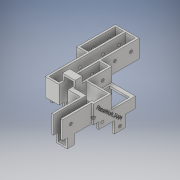
# Autodesk Inventor part: Gear Train Chassis Version 2
Saved by Autodesk Inventor 2017 (Build 210142000, 142)
## iProperties
Created: 2019-11-21
Part Number: Gear Train Chassis Version 2
Material: Generic
Document SubType Name: Modeling
Designer: asadb
Density: 1 g/cm^3
Appearance: Default
Author: asadb
Autodesk Inventor part; units mm, degrees
note: some values were not read from the file. Chosen so that the rebuilt part matches the saved one: direction of "Emboss1".
ref_plane "YZ Plane" through (0, 0, 0) normal (1, 0, 0) x (0, 1, 0)
sketch "Sketch1" plane through (0, 0, 0) normal (0, 1, 0) x (-1, 0, 0)
  line L0 (0, 84.0002) -> (-10, 84.0002)
  line L1 (-10, 84.0002) -> (-10, 76)
  line L2 (-10, 76) -> (-74.5, 76)
  line L3 (-74.5, 76) -> (-74.5, 65.5)
  line L4 (-74.5, 65.5) -> (-91, 65.5)
  line L5 (-91, 65.5) -> (-91, 36)
  line L6 (-91, 36) -> (-69, 36)
  line L7 (-69, 36) -> (-69, 6)
  line L8 (-69, 6) -> (-25, 6)
  line L9 (-25, 6) -> (-25, 0)
  line L10 (-25, 0) -> (0, 0)
  line L11 (0, 16.033) -> (32, 16.033)
  line L12 (32, 16.033) -> (32, 2.033)
  line L13 (32, 2.033) -> (0, 2.033)
  line L14 (0, 0) -> (0, 2.033)
  line L15 (0, 16.033) -> (0, 84.0002)
  point P0 (0, 0)
  point P1 (0, 0)
  dimension "d0" = 84.0002
  dimension "d1" = 25
  dimension "d2" = 6
  dimension "d3" = 44
  dimension "d4" = 30
  dimension "d5" = 29.5
  dimension "d6" = 22
  dimension "d7" = 16.5
  dimension "d8" = 64.5
  dimension "d9" = 76
  dimension "d17" = 2.033
  dimension "d18" = 14
  dimension "d19" = 32
  dimension "d20" = 2.033
  dimension "d21" = 32
  dimension "d22" = 84.0002
  constraints: 32 end point, 13 perpendicular, 2 vertical, 1 horizontal, 1 parallel, 1 other
  measures "d0" distance of L0.start L10.end
  measures "d1" distance of L9.end L10.end
  measures "d2" distance of L9.end L8.end
  measures "d3" distance of L7.end L8.end
  measures "d4" distance of L6.end L7.end
  measures "d5" distance of L4.end L5.end
  measures "d6" distance of L5.end L6.end
  measures "d7" distance of L3.end L4.end
  measures "d8" distance of L1.end L2.end
  measures "d9" distance between parallel lines of L2 L10
  measures "d17" distance from line of point (0, 0) L13
  measures "d18" distance of L11.end L12.end
  measures "d19" distance of L11.start L11.end
  measures "d20" distance of L10.end L13.end
  measures "d21" distance from line of point (0, 0) L12
  measures "d22" distance from line of point (0, 0) L0
surface extrude "ExtrusionSrf1" sketch "Sketch1" along normal blind 30 shown no curves L1 L2 L3 L4 L5 L6 L7 L8 L9 L10 L14 L13 L12 L11 L15 L0
sketch "Sketch2" plane through (0, 0, 0) normal (0, 1, 0) x (-1, 0, 0)
  line L0 (-74.5, 76) -> (-74.5, 65.5) projected
  line L1 (-0.8, 0.8) -> (-21.1, 0.8)
  line L2 (-21.1, 0.8) -> (-21.1, 26.9714)
  line L3 (-21.1, 26.9714) -> (-47.7, 26.9714)
  line L4 (-47.7, 26.9714) -> (-47.7, 39.0002)
  line L5 (-74.5, 65.5) -> (-91, 65.5) projected
  line L6 (-90.2, 65.5) -> (-74.5, 65.5)
  line L7 (-25, 0) -> (0, 0) projected
  line L8 (-0.8, 15.233) -> (31.2, 15.233)
  line L9 (31.2, 2.833) -> (-0.8, 2.833)
  line L10 (-0.8, 2.833) -> (-0.8, 0.8)
  line L11 (32, 16.033) -> (0, 16.033) projected
  line L12 (32, 2.033) -> (32, 16.033) projected
  line L13 (0, 2.033) -> (32, 2.033) projected
  line L14 (0, 0) -> (0, 2.033) projected
  line L15 (-25, 6) -> (-25, 0) projected
  line L16 (0, 16.033) -> (0, 84.0002) projected
  line L17 (5.242, 5.033) -> (29, 5.033)
  line L18 (29, 13.033) -> (6.042, 13.033)
  line L19 (-18.9, 3) -> (-3.8, 3)
  line L20 (-18.9, 20.868) -> (-18.9, 3)
  line L21 (5.242, 5.033) -> (-3.8, 5.033)
  line L22 (6.042, 13.033) -> (-5.6, 13.033)
  line L23 (-3.8, 3) -> (-3.8, 5.033)
  line L24 (-5.6, 13.033) -> (-5.6, 20.868)
  line L25 (31.2, 15.233) -> (31.2, 13.033)
  line L26 (31.2, 5.033) -> (31.2, 2.833)
  line L27 (29, 13.033) -> (31.2, 13.033)
  line L28 (29, 5.033) -> (31.2, 5.033)
  line L29 (23, 13.033) -> (23, 5.033) construction
  line L30 (-10.9, 3) -> (-10.9, 52.2501) construction
  line L31 (-81, 65.5) -> (-81, 76) construction
  line L32 (-91, 65.5) -> (-91, 36) construction
  line L33 (-88, 63.3) -> (-63.0024, 63.3)
  line L34 (-63.0024, 39.0002) -> (-88, 39.0002)
  line L35 (-91, 36) -> (-69, 36) construction
  line L36 (-45.5, 39.0002) -> (-45.5, 29.1714)
  line L37 (-45.5, 29.1714) -> (-21.6831, 29.1714)
  line L38 (-18.9, 26.9714) -> (-18.9, 20.868)
  line L39 (-37.5, 52.2501) -> (-37.5, 29.1714) construction
  line L40 (-30.5, 29.1714) -> (-30.5, 52.2501) construction
  line L41 (0, 84.0002) -> (-10, 84.0002) projected
  line L42 (-3, 41.2002) -> (-88, 41.2002)
  line L43 (-81, 65.5) -> (-81, 41.2002) construction
  line L44 (-81, 39.0002) -> (-81, 39.0002) construction
  line L45 (-63, 63.3) -> (-63, 41.2002) construction
  line L46 (-45.5, 39.0002) -> (-45.5, 39.0002) construction
  line L47 (-90.2, 39.0002) -> (-90.2, 65.5)
  line L48 (-88, 39.0002) -> (-90.2, 39.0002)
  line L49 (-3, 52.2501) -> (-3, 41.2002)
  line L50 (-5.6, 26.9714) -> (-5.6, 20.868)
  line L51 (-69, 36) -> (-69, 6) projected
  line L52 (-3, 39.0002) -> (-0.8, 39.0002)
  line L53 (-21.6831, 29.1714) -> (-3, 29.1714)
  line L54 (-18.9, 26.9714) -> (-5.6, 26.9714)
  line L55 (-3, 29.1714) -> (-0.8, 29.1714)
  line L56 (-0.8, 29.1714) -> (-0.8, 15.233)
  line L57 (-69, 6) -> (-25, 6) projected
  line L58 (-88, 52.2501) -> (-3, 52.2501)
  line L59 (-49, 63.3) -> (-49, 54.4501)
  line L60 (-46.8, 63.3) -> (-46.8, 54.4501)
  line L61 (-46.8, 63.3) -> (-46.8, 65.5)
  line L62 (-74.5, 65.5) -> (-46.8, 65.5)
  line L63 (-63, 63.3) -> (-49, 63.3)
  line L64 (-0.8, 54.4501) -> (-0.8, 39.0002)
  line L65 (-3, 54.4501) -> (-0.8, 54.4501)
  line L66 (-88, 54.4501) -> (-49, 54.4501)
  line L67 (-46.8, 54.4501) -> (-3, 54.4501)
  line L68 (-88, 41.2002) -> (-88, 52.2501)
  line L69 (-88, 54.4501) -> (-88, 63.3)
  line L70 (-3, 39.0002) -> (-45.5, 39.0002)
  line L71 (-47.7, 39.0002) -> (-88, 39.0002)
  dimension "d14" = 0.8
  dimension "d23" = 0.8
  dimension "d25" = 0.8
  dimension "d26" = 0.8
  dimension "d33" = 3
  dimension "d35" = 3
  dimension "d36" = 3
  dimension "d37" = 5.6
  dimension "d38" = 3
  dimension "d43" = 0.8
  dimension "d44" = 0.8
  dimension "d45" = 9
  dimension "d53" = 10
  dimension "d60" = 2.2
  dimension "d65" = 2.2
  dimension "d67" = 26.6
  dimension "d68" = 30.5
  dimension "d71" = 0.8
  dimension "d74" = 8
  dimension "d75" = 8
  dimension "d76" = 2.2
  dimension "d79" = 21.3
  dimension "d80" = 20.9714
  dimension "d82" = 2.2
  dimension "d83" = 14
  dimension "d84" = 18
  dimension "d85" = 2.2
  dimension "d86" = 0.8
  dimension "d87" = 29.5501
  dimension "d88" = 2.2
  dimension "d89" = 4.8
  dimension "d90" = 2.2
  dimension "d91" = 2.2
  dimension "d92" = 2.2
  dimension "d93" = 2.2
  dimension "d94" = 2.2
  dimension "d95" = 40.3
  dimension "d96" = 85
  dimension "d97" = 42.5
  dimension "d98" = 11.0499
  dimension "d99" = 2.2
  constraints: 116 end point, 36 perpendicular, 20 point on line, 12 parallel, 8 horizontal, 5 collinear, 3 vertical
  measures "d14" distance between parallel lines of L7 L1
  measures "d23" distance between parallel lines of L11 L8
  measures "d25" distance between parallel lines of L13 L9
  measures "d26" distance between parallel lines of L14 L10
  measures "d33" distance between parallel lines of L7 L19
  measures "d35" distance between parallel lines of L11 L18
  measures "d36" distance between parallel lines of L13 L17
  measures "d37" distance between parallel lines of L16 L24
  measures "d38" distance between parallel lines of L10 L23
  measures "d43" distance between parallel lines of L12 L25
  measures "d44" distance between parallel lines of L12 L26
  measures "d45" distance between parallel lines of L12 L29
  measures "d53" distance between parallel lines of L32 L31
  measures "d60" distance between parallel lines of L6 L33
  measures "d65" distance between parallel lines of L4 L36
  measures "d67" distance between parallel lines of L39 L30
  measures "d68" distance between parallel lines of L16 L40
  measures "d71" distance from line of L5.end L47
  measures "d74" distance between parallel lines of L36 L39
  measures "d75" distance between parallel lines of L38 L30
  measures "d76" distance between parallel lines of L2 L20
  measures "d79" distance between parallel lines of L51 L4
  measures "d80" distance between parallel lines of L57 L3
  measures "d82" distance between parallel lines of L60 L59
  measures "d83" distance between parallel lines of L45 L59
  measures "d84" distance between parallel lines of L43 L45
  measures "d85" distance between parallel lines of L49 L64
  measures "d86" distance between parallel lines of L16 L64
  measures "d87" distance between parallel lines of L41 L65
  measures "d88" distance between parallel lines of L3 L37
  measures "d89" distance between parallel lines of L50 L56
  measures "d90" distance between parallel lines of L58 L66
  measures "d91" distance between parallel lines of L47 L69
  measures "d92" distance between parallel lines of L71 L42
  measures "d93" distance between parallel lines of L70 L42
  measures "d94" distance between parallel lines of L58 L67
  measures "d95" distance of L4.end L48.start
  measures "d96" distance of L42.start L42.end
  measures "d97" distance of L52.start L36.start
  measures "d98" distance of L42.end L58.start
  measures "d99" distance between parallel lines of L53 L54
extrude "Extrusion1" add sketch "Sketch2" along normal blind 20
sketch "Sketch3" plane through (0, 0, 0) normal (0, -1, 0) x (1, 0, 0)
  line L0 (88, 63.3) -> (49, 63.3)
  line L1 (49, 63.3) -> (49, 54.4501)
  line L2 (49, 54.4501) -> (88, 54.4501)
  line L3 (88, 54.4501) -> (88, 63.3)
  line L4 (46.8, 65.5) -> (90.2, 65.5) projected
  line L5 (90.2, 65.5) -> (90.2, 39.0002) projected
  line L6 (3, 52.2501) -> (88, 52.2501) projected
  line L7 (46.8, 54.4501) -> (46.8, 65.5) projected
  point P0 (0, 0)
  dimension "d102" = 2.2
  dimension "d103" = 2.2
  dimension "d104" = 2.2
  dimension "d105" = 2.2
  constraints: 8 end point, 2 parallel, 1 horizontal, 1 perpendicular
  measures "d102" distance between parallel lines of L4 L0
  measures "d103" distance between parallel lines of L5 L3
  measures "d104" distance between parallel lines of L6 L2
  measures "d105" distance between parallel lines of L7 L1
extrude "Extrusion2" cut sketch "Sketch3" against normal blind 20
ref_plane "Work Plane1" through (10.9, 0, 29.1714) normal (-1, 0, 0) x (0, 0, 1)
sketch "Sketch4" plane through (10.9, 0, 29.1714) normal (-1, 0, 0) x (0, 0, 1)
  line L0 (9.6527, -4.76) -> (-0.0402, -4.76) construction
  line L1 (0, 0) -> (0, 20) construction
  line L2 (9.8288, 20) -> (25.2787, 20) construction
  line L3 (-13.9384, 0) -> (0, 0) construction
  line L4 (10.9288, -5.86) -> (-1.1, -5.86)
  line L5 (9.8288, 0) -> (9.8288, 20) projected
  line L6 (10.9288, -5.86) -> (10.9288, 0)
  line L7 (-1.1, -5.86) -> (-1.1, 0)
  point P0 (-29.1714, 0)
  point P1 (4.9145, 22.24)
  dimension "d109" = 4.9145
  dimension "d110" = 2.24
  dimension "d111" = 27
  dimension "d112" = 9.6929
  dimension "d113" = 4.9547
  dimension "d114" = 1.1
  dimension "d115" = 1.1
  dimension "d116" = 28.1
  constraints: 8 end point, 1 horizontal, 1 parallel, 1 perpendicular, 1 point on line, 1 vertical
  measures "d109" distance from line of L1 point (4.915, 22.24)
  measures "d110" distance from line of L2 point (4.915, 22.24)
  measures "d111" distance from line of point (4.915, 22.24) L0
  measures "d112" distance of L0.start L0.end
  measures "d113" horizontal distance of L0.end point (4.915, 22.24)
  measures "d114" horizontal distance of L1.start L4.end
  measures "d115" distance from line of L5 L4.start
  measures "d116" distance from line of point (4.915, 22.24) L4
sketch "Sketch6" plane through (0, 0, 0) normal (0, -1, 0) x (1, 0, 0)
  line L0 (14.8, 41.2002) -> (6.8, 41.2002)
  line L1 (6.8, 41.2002) -> (6.8, 39.0002)
  line L2 (6.8, 39.0002) -> (14.8, 39.0002)
  line L3 (14.8, 39.0002) -> (14.8, 41.2002)
  line L4 (88, 41.2002) -> (3, 41.2002) projected
  line L5 (0.8, 39.0002) -> (0.8, 54.4501) projected
  point P0 (0, 0)
  dimension "d117" = 2.2
  dimension "d118" = 0
  dimension "d119" = 8
  dimension "d120" = 6
  constraints: 8 end point, 2 parallel, 1 horizontal, 1 perpendicular
  measures "d117" distance of L1.end L0.end
  measures "d118" distance between parallel lines of L4 L0
  measures "d119" distance between parallel lines of L1 L3
  measures "d120" distance between parallel lines of L5 L1
sweep "Sweep1" add profiles "Sketch6" path "Sketch4" path curves L6 L4 L7
sketch "Sketch7" plane through (0.8, 0, 2.833) normal (0, 0, -1) x (-1, 0, 0)
  line L0 (32, 0) -> (32, 20) projected
  line L1 (32, 0) -> (-3, 0) projected
  point P0 (0.8, 0)
  point P1 (23, 8.5)
  dimension "d123" = 9
  dimension "d124" = 8.5
  measures "d123" distance from line of point (23, 8.5) L0
  measures "d124" distance from line of L1 point (23, 8.5)
ref_plane "Work Plane2" through (-22.2, 0, 13.033) normal (-1, 0, 0) x (0, 0, 1)
sketch "Sketch8" plane through (-22.2, 0, 13.033) normal (-1, 0, 0) x (0, 0, 1)
  line L0 (0, 0) -> (0, 20) projected
  line L1 (0, 0) -> (2.2, 0) projected
  line L2 (1.1, 29.5) -> (-9.1, 29.5)
  line L3 (-10.2, 0) -> (-10.2, 20) projected
  line L4 (2.2, 0) -> (2.2, 20) projected
  line L5 (1.1, 29.5) -> (1.1, 20)
  line L6 (0, 20) -> (2.2, 20) projected
  line L7 (-9.1, 29.5) -> (-9.1, 20)
  line L8 (-8, 20) -> (-10.033, 20) projected
  line L9 (-10.2, 20) -> (-8, 20) projected
  point P0 (-13.033, 0)
  point P1 (-4, 8.5)
  dimension "d126" = 4
  dimension "d127" = 8.5
  dimension "d128" = 1.1
  dimension "d129" = 1.1
  dimension "d130" = 21
  constraints: 6 end point, 2 perpendicular, 1 horizontal, 1 midpoint, 1 point on line
  measures "d126" distance from line of L0 point (-4, 8.5)
  measures "d127" distance from line of L1 point (-4, 8.5)
  measures "d128" distance from line of L3 L2.end
  measures "d129" distance from line of L4 L2.start
  measures "d130" distance from line of point (-4, 8.5) L2
sketch "Sketch9" plane through (0, 20, 0) normal (0, 1, 0) x (1, 0, 0)
  line L0 (-26.2, -15.233) -> (-18.2, -15.233)
  line L1 (-18.2, -15.233) -> (-18.2, -13.033)
  line L2 (-18.2, -13.033) -> (-26.2, -13.033)
  line L3 (-26.2, -13.033) -> (-26.2, -15.233)
  line L4 (-31.2, -15.233) -> (0.8, -15.233) projected
  line L5 (5.6, -13.033) -> (-31.2, -13.033) projected
  line L6 (-31.2, -13.033) -> (-31.2, -15.233) projected
  point P0 (0, 0)
  dimension "d131" = 0
  dimension "d132" = 0
  dimension "d134" = 8
  dimension "d135" = 5
  constraints: 8 end point, 2 parallel, 1 horizontal, 1 perpendicular
  measures "d131" distance between parallel lines of L4 L0
  measures "d132" distance between parallel lines of L5 L2
  measures "d134" distance of L1.end L2.end
  measures "d135" distance between parallel lines of L3 L6
sweep "Sweep2" add profiles "Sketch9" path "Sketch8" path curves L5 L2 L7 contours L3 L2 L1 L0
sketch "Sketch10" plane through (90.2, 0, 39.0002) normal (0, 0, -1) x (-1, 0, 0)
  line L0 (0, 0) -> (0, 20) projected
  line L1 (0, 0) -> (42.5, 0) projected
  line L2 (44.7, 0) -> (75.4, 0) projected
  point P0 (90.2, 0)
  point P1 (9.2, 8.5)
  point P2 (27.2, 8.5)
  point P3 (52.7, 8.5)
  dimension "d138" = 9.2
  dimension "d139" = 8.5
  dimension "d140" = 18
  dimension "d141" = 8.5
  dimension "d143" = 25.5
  dimension "d144" = 8.5
  measures "d138" distance from line of L0 point (9.2, 8.5)
  measures "d139" distance from line of L1 point (9.2, 8.5)
  measures "d140" distance of point (9.2, 8.5) point (27.2, 8.5)
  measures "d141" distance from line of L1 point (27.2, 8.5)
  measures "d143" distance of point (27.2, 8.5) point (52.7, 8.5)
  measures "d144" distance from line of L2 point (52.7, 8.5)
hole "Hole1" at (63, 8.5, 39.0002) at (81, 8.5, 39.0002) direction (0, 0, 1) diameter 3.302 end through all
sketch "Sketch11" plane through (47.7, 0, 26.9714) normal (0, 0, -1) x (-1, 0, 0)
  line L0 (32.9, 0) -> (2.2, 0) projected
  line L1 (-42.5, 0) -> (-42.5, 20) projected
  point P0 (47.7, 0)
  point P1 (10.2, 8.5)
  dimension "d152" = 8.5
  dimension "d153" = 52.7
  measures "d152" distance from line of L0 point (10.2, 8.5)
  measures "d153" distance from line of L1 point (10.2, 8.5)
hole "Hole2" at (37.5, 8.5, 26.9714) direction (0, 0, 1) diameter 3.302 end through all
hole "Hole3" at (-22.2, 8.5, 2.833) direction (0, 0, 1) diameter 3.302 end through all
sketch "Sketch12" plane through (0, 20, 0) normal (0, 1, 0) x (1, 0, 0)
  line L0 (6.8, -52.2501) -> (14.8, -52.2501)
  line L1 (14.8, -52.2501) -> (14.8, -54.4501)
  line L2 (14.8, -54.4501) -> (6.8, -54.4501)
  line L3 (6.8, -54.4501) -> (6.8, -52.2501)
  line L4 (3, -52.2501) -> (88, -52.2501) projected
  line L5 (0.8, -39.0002) -> (0.8, -54.4501) projected
  line L6 (6.8, -39.0002) -> (14.8, -39.0002)
  line L7 (14.8, -39.0002) -> (14.8, -41.2002)
  line L8 (14.8, -41.2002) -> (6.8, -41.2002)
  line L9 (6.8, -41.2002) -> (6.8, -39.0002)
  line L10 (6.8, -26.9714) -> (14.8, -26.9714)
  line L11 (14.8, -26.9714) -> (14.8, -29.1714)
  line L12 (14.8, -29.1714) -> (6.8, -29.1714)
  line L13 (6.8, -29.1714) -> (6.8, -26.9714)
  line L14 (6.8, -0.8) -> (14.8, -0.8)
  line L15 (14.8, -0.8) -> (14.8, -3)
  line L16 (14.8, -3) -> (6.8, -3)
  line L17 (6.8, -3) -> (6.8, -0.8)
  line L18 (3, -41.2002) -> (88, -41.2002) construction
  line L19 (18.9, -26.9714) -> (5.6, -26.9714) construction
  line L20 (3.8, -3) -> (18.9, -3) construction
  point P0 (0, 0)
  dimension "d168" = 8
  dimension "d169" = 2.2
  dimension "d170" = 0
  dimension "d171" = 6
  dimension "d172" = 8
  dimension "d173" = 2.2
  dimension "d174" = 8
  dimension "d175" = 2.2
  dimension "d176" = 8
  dimension "d177" = 2.2
  dimension "d178" = 0
  dimension "d179" = 0
  dimension "d180" = 0
  constraints: 32 end point, 8 parallel, 4 horizontal, 4 perpendicular, 3 collinear
  measures "d168" distance of L1.end L2.end
  measures "d169" distance of L0.end L1.end
  measures "d170" distance between parallel lines of L4 L0
  measures "d171" distance between parallel lines of L5 L3
  measures "d172" distance of L7.end L8.end
  measures "d173" distance of L6.end L7.end
  measures "d174" distance of L11.end L12.end
  measures "d175" distance of L10.end L11.end
  measures "d176" distance of L15.end L16.end
  measures "d177" distance of L14.end L15.end
  measures "d178" distance between parallel lines of L18 L8
  measures "d179" distance between parallel lines of L19 L10
  measures "d180" distance between parallel lines of L20 L16
extrude "Extrusion3" add sketch "Sketch12" along normal blind 7.5
sketch "Sketch15" plane through (0.8, 0, 54.4501) normal (0, 0, 1) x (1, 0, 0)
  circle A0 centre (36.7, 8.5) radius 1.651 construction
  line L0 (36.7, 8.5) -> (10.0336, 22.2441) construction
  line L1 (36.7, 8.5) -> (66.7, 8.5) construction
  point P0 (-0.8, 0)
  dimension "d203" = 30
  dimension "d204" = 152.733
  constraints: 4 end point, 1 coincident, 1 equal length, 1 horizontal
  measures "d203" distance of L0.start L0.end
  measures "d204" angle of L1 L0
hole "Hole6" at (10.8336, 22.2441, 54.4501) direction (0, 0, -1) diameter 3.302 end through all
sketch "Sketch16" plane through (21.1, 0, 0.8) normal (0, 0, -1) x (-1, 0, 0)
  circle A0 centre (10.2664, 22.2441) radius 1.651 construction
  line L0 (10.2664, 22.2441) -> (19.3486, 13.6555) construction
  line L1 (10.2664, 22.2441) -> (22.7664, 22.2441) construction
  circle A1 centre (43.3, 8.5) radius 1.651 projected
  point P0 (21.1, 0)
  dimension "d212" = 12.5
  dimension "d257" = 24.5
  constraints: 4 end point, 1 coincident, 1 equal length, 1 horizontal
  measures "d212" distance of L0.start L0.end
  measures "d257" distance of A1.centre point (19.349, 13.655)
hole "Hole7" at (1.7514, 13.6555, 0.8) direction (0, 0, 1) diameter 3.302 depth 16.533 tip angle 118
sketch "Sketch17" plane through (21.1, 0, 0.8) normal (0, 0, -1) x (-1, 0, 0)
  circle A0 centre (-16.4, 8.5) radius 1.651 construction
  line L0 (-16.4, 8.5) -> (-9.4008, 35.9992) construction
  line L1 (-16.4, 8.5) -> (11.9759, 8.5) construction
  circle A1 centre (10.2664, 22.2441) radius 1.651 construction
  point P0 (21.1, 0)
  dimension "d221" = 75.72
  dimension "d222" = 24
  constraints: 4 end point, 1 coincident, 1 equal length, 1 horizontal
  measures "d221" angle of L1 L0
  measures "d222" distance of A1.centre L0.end
sketch "Sketch18" plane through (14.8, 20, 3) normal (1, 0, 0) x (0, 0, -1)
  line L0 (2.2, 0) -> (2.2, 7.5) projected
  line L1 (0, 0) -> (0, 7.5) projected
  line L2 (2.2, 0) -> (0, 0)
  line L3 (0, 0) -> (0, 7.5)
  line L4 (0, 7.5) -> (2.2, 7.5)
  line L5 (2.2, 7.5) -> (2.2, 0)
  line L6 (-23.9714, 0) -> (-26.1714, 0) projected
  line L7 (-26.1714, 0) -> (-26.1714, 7.5) projected
  line L8 (-23.9714, 0) -> (-26.1714, 0)
  line L9 (-26.1714, 0) -> (-26.1714, 7.5)
  line L10 (-26.1714, 7.5) -> (-23.9714, 7.5)
  line L11 (-23.9714, 7.5) -> (-23.9714, 0)
  point P0 (3, -20)
  constraints: 16 end point, 4 parallel, 2 horizontal, 2 perpendicular
extrude "Extrusion4" add sketch "Sketch18" along normal up to surface (32.9 mm away)
sketch "Sketch19" plane through (21.1, 0, 26.9714) normal (1, 0, 0) x (0, 0, -1)
  line L0 (23.9714, 20) -> (26.1714, 20) projected
  line L1 (0, 0) -> (0, 20) projected
  line L2 (26.1714, 20) -> (0, 20)
  line L3 (0, 20) -> (0, 17.8)
  line L4 (0, 17.8) -> (26.1714, 17.8)
  line L5 (26.1714, 17.8) -> (26.1714, 20)
  point P0 (26.9714, 0)
  dimension "d225" = 2.2
  constraints: 8 end point, 2 parallel, 1 horizontal, 1 perpendicular, 1 point on line
  measures "d225" distance of L3.end L2.end
extrude "Extrusion5" add sketch "Sketch19" along normal up to surface (26.6 mm away)
sketch "Sketch20" plane through (0, 27.5, 0) normal (0, 1, 0) x (1, 0, 0)
  line L0 (6.8, -0.8) -> (47.7, -0.8) projected
  line L1 (6.8, -3) -> (47.7, -3) projected
  line L2 (24.2, -0.8) -> (36.2, -0.8)
  line L3 (36.2, -0.8) -> (36.2, -3)
  line L4 (36.2, -3) -> (24.2, -3)
  line L5 (24.2, -3) -> (24.2, -0.8)
  line L6 (47.7, -3) -> (47.7, -0.8) projected
  line L7 (6.8, -29.1714) -> (47.7, -29.1714) projected
  line L8 (24.2, -29.1714) -> (36.2, -29.1714)
  line L9 (36.2, -29.1714) -> (36.2, -26.9714)
  line L10 (36.2, -26.9714) -> (24.2, -26.9714)
  line L11 (24.2, -26.9714) -> (24.2, -29.1714)
  point P0 (0, 0)
  dimension "d228" = 12
  dimension "d229" = 11.5
  dimension "d230" = 12
  dimension "d231" = 2.2
  dimension "d232" = 0
  constraints: 16 end point, 4 parallel, 3 point on line, 2 horizontal, 2 perpendicular
  measures "d228" distance between parallel lines of L3 L5
  measures "d229" distance between parallel lines of L6 L3
  measures "d230" distance of L10.end L9.end
  measures "d231" distance of L9.end L8.end
  measures "d232" distance between parallel lines of L11 L5
extrude "Extrusion6" add sketch "Sketch20" along normal blind 13 contours L0 L3 L1 L5 | L11 L10 L9 L7
hole "Hole8" at (30.5008, 35.9992, 0.8) direction (0, 0, 1) diameter 3.302 end through all
sketch "Sketch21" plane through (47.7, 0, 39.0002) normal (1, 0, 0) x (0, 0, -1)
  line L0 (36.0002, 20) -> (36.0002, 27.5) projected
  line L1 (38.2002, 17.8) -> (12.0288, 17.8) projected
  line L2 (36.0002, 20) -> (12.0288, 20)
  line L3 (12.0288, 20) -> (12.0288, 17.8)
  line L4 (12.0288, 17.8) -> (36.0002, 17.8)
  line L5 (36.0002, 17.8) -> (36.0002, 20)
  point P0 (39.0002, 0)
  constraints: 8 end point, 2 parallel, 1 horizontal, 1 perpendicular
extrude "Extrusion7" cut sketch "Sketch21" against normal blind 29
sketch "Sketch23" plane through (47.7, 0, 39.0002) normal (1, 0, 0) x (0, 0, -1)
  line L0 (38.2002, 27.5) -> (38.2002, 17.8) projected
  line L1 (12.0288, 0) -> (12.0288, 17.8) projected
  line L2 (38.2002, 17.8) -> (12.0288, 17.8)
  line L3 (12.0288, 17.8) -> (12.0288, 15.6)
  line L4 (12.0288, 15.6) -> (38.2002, 15.6)
  line L5 (38.2002, 15.6) -> (38.2002, 17.8)
  point P0 (39.0002, 0)
  dimension "d245" = 2.2
  constraints: 8 end point, 2 parallel, 1 horizontal, 1 perpendicular, 1 point on line
  measures "d245" distance of L3.end L2.end
extrude "Extrusion8" add sketch "Sketch23" against normal blind 4.4167
sketch "Sketch24" plane through (21.1, 17.8, 0.8) normal (0, -1, 0) x (1, 0, 0)
  line L0 (0, 0) -> (0, 2.2) projected
  line L1 (22.1833, 0) -> (22.1833, 26.1714) projected
  line L2 (0, 0) -> (22.1833, 0)
  line L3 (22.1833, 0) -> (22.1833, 2.2)
  line L4 (22.1833, 2.2) -> (0, 2.2)
  line L5 (0, 2.2) -> (0, 0)
  point P0 (-21.1, -0.8)
  dimension "d248" = 2.2
  constraints: 8 end point, 2 parallel, 1 horizontal, 1 perpendicular, 1 point on line
  measures "d248" distance of L3.end L2.end
extrude "Extrusion9" add sketch "Sketch24" along normal blind 2.2
sketch "Sketch25" plane through (21.1, 0, 26.9714) normal (1, 0, 0) x (0, 0, -1)
  line L0 (0, 0) -> (0, 17.8) projected
  line L1 (0, 17.8) -> (2.2, 17.8)
  line L2 (2.2, 17.8) -> (2.2, 15.6)
  line L3 (2.2, 15.6) -> (0, 15.6)
  line L4 (0, 15.6) -> (0, 17.8)
  point P0 (26.9714, 0)
  dimension "d251" = 2.2
  dimension "d252" = 2.2
  constraints: 8 end point, 2 parallel, 1 horizontal, 1 perpendicular
  measures "d251" distance of L2.end L3.end
  measures "d252" distance of L1.end L2.end
extrude "Extrusion10" add sketch "Sketch25" along normal up to surface (22.1833 mm away)
sketch "Sketch26" plane through (21.1, 0, 0.8) normal (0, 0, -1) x (-1, 0, 0)
  line L0 (15.1438, 3.2996) -> (-7.5912, 23.6414) construction
  line L1 (-7.5912, 23.6414) -> (-0.9379, 31.0775) construction
  line L2 (-0.9379, 31.0775) -> (21.7972, 10.7357) construction
  line L3 (21.7972, 10.7357) -> (15.1438, 3.2996) construction
  spline S0 degree 2 poles (14.0385, 5.9137) (14.1898, 6.0828) (14.5826, 6.2794) (14.7849, 6.2886) knots 0 0 0 1 2 2 2
  spline S1 degree 2 poles (14.7849, 6.2886) (15.0394, 6.3008) (15.528, 6.111) (15.807, 5.8613) knots 0 0 0 1 2 2 2
  line L4 (15.807, 5.8613) -> (16.1008, 5.5984)
  line L5 (16.1008, 5.5984) -> (16.9708, 6.5708)
  line L6 (16.9708, 6.5708) -> (17.3174, 6.2606)
  line L7 (17.3174, 6.2606) -> (14.9836, 3.6522)
  line L8 (14.9836, 3.6522) -> (14.3284, 4.2385)
  spline S2 degree 2 poles (14.3284, 4.2385) (14.0959, 4.4466) (13.8384, 4.8139) (13.7913, 5.0121) knots 0 0 0 1 2 2 2
  spline S3 degree 2 poles (13.7913, 5.0121) (13.7343, 5.242) (13.8437, 5.696) (14.0385, 5.9137) knots 0 0 0 1 2 2 2
  spline S4 degree 2 poles (14.4094, 5.6009) (14.2883, 5.4656) (14.2036, 5.1837) (14.2419, 5.0352) knots 0 0 0 1 2 2 2
  spline S5 degree 2 poles (14.2419, 5.0352) (14.2752, 4.9065) (14.4553, 4.6654) (14.6181, 4.5198) knots 0 0 0 1 2 2 2
  line L9 (14.6181, 4.5198) -> (14.9055, 4.2626)
  line L10 (14.9055, 4.2626) -> (15.836, 5.3025)
  line L11 (15.836, 5.3025) -> (15.5993, 5.5143)
  spline S6 degree 2 poles (15.5993, 5.5143) (15.3879, 5.7035) (15.0674, 5.8684) (14.9034, 5.8553) knots 0 0 0 1 2 2 2
  spline S7 degree 2 poles (14.9034, 5.8553) (14.7552, 5.8471) (14.5209, 5.7256) (14.4094, 5.6009) knots 0 0 0 1 2 2 2
  line L12 (15.0282, 8.3088) -> (15.358, 8.0138)
  line L13 (15.358, 8.0138) -> (12.9202, 5.2892)
  line L14 (12.9202, 5.2892) -> (12.5904, 5.5842)
  line L15 (12.5904, 5.5842) -> (15.0282, 8.3088)
  spline S8 degree 2 poles (13.7342, 9.5465) (14.2034, 9.1267) (14.2483, 8.1389) (13.8133, 7.6528) knots 0 0 0 1 2 2 2
  spline S9 degree 2 poles (13.8133, 7.6528) (13.3859, 7.1751) (12.3781, 7.0568) (11.9743, 7.418) knots 0 0 0 1 2 2 2
  spline S10 degree 2 poles (11.9743, 7.418) (11.7926, 7.5807) (11.606, 7.9379) (11.6027, 8.1426) knots 0 0 0 1 2 2 2
  spline S11 degree 2 poles (11.6027, 8.1426) (11.5972, 8.3492) (11.7745, 8.7728) (11.9845, 9.0074) knots 0 0 0 1 2 2 2
  line L16 (11.9845, 9.0074) -> (12.1452, 9.1871)
  line L17 (12.1452, 9.1871) -> (13.5001, 7.9748)
  spline S12 degree 2 poles (13.5001, 7.9748) (13.8046, 8.3151) (13.7856, 8.983) (13.4812, 9.2553) knots 0 0 0 1 2 2 2
  spline S13 degree 2 poles (13.4812, 9.2553) (13.3734, 9.3517) (13.1206, 9.4904) (13.002, 9.528) knots 0 0 0 1 2 2 2
  spline S14 degree 2 poles (13.002, 9.528) (12.8754, 9.5651) (12.6867, 9.6008) (12.6162, 9.6029) knots 0 0 0 1 2 2 2
  line L18 (12.6162, 9.6029) -> (12.5972, 9.62)
  line L19 (12.5972, 9.62) -> (12.9187, 9.9793)
  spline S15 degree 2 poles (12.9187, 9.9793) (12.9966, 9.9515) (13.2304, 9.8641) (13.3151, 9.8226) knots 0 0 0 1 2 2 2
  spline S16 degree 2 poles (13.3151, 9.8226) (13.4348, 9.7649) (13.6158, 9.6525) (13.7342, 9.5465) knots 0 0 0 1 2 2 2
  spline S17 degree 2 poles (12.2414, 8.6481) (12.1265, 8.5111) (12.0075, 8.2675) (12.0017, 8.1547) knots 0 0 0 1 2 2 2
  spline S18 degree 2 poles (12.0017, 8.1547) (11.9926, 8.0297) (12.1023, 7.7907) (12.2354, 7.6716) knots 0 0 0 1 2 2 2
  spline S19 degree 2 poles (12.2354, 7.6716) (12.3665, 7.5543) (12.6204, 7.468) (12.7645, 7.476) knots 0 0 0 1 2 2 2
  spline S20 degree 2 poles (12.7645, 7.476) (12.9085, 7.488) (13.1529, 7.608) (13.2751, 7.7233) knots 0 0 0 1 2 2 2
  line L20 (13.2751, 7.7233) -> (12.2414, 8.6481)
  spline S21 degree 2 poles (11.3806, 11.1995) (11.4472, 11.1931) (11.6771, 11.1778) (11.7688, 11.1528) knots 0 0 0 1 2 2 2
  spline S22 degree 2 poles (11.7688, 11.1528) (11.8971, 11.1217) (12.1034, 11.0247) (12.2513, 10.8923) knots 0 0 0 1 2 2 2
  spline S23 degree 2 poles (12.2513, 10.8923) (12.3718, 10.7845) (12.5082, 10.4988) (12.5169, 10.3426) knots 0 0 0 1 2 2 2
  spline S24 degree 2 poles (12.5169, 10.3426) (12.5232, 10.1923) (12.4065, 9.8705) (12.2893, 9.7394) knots 0 0 0 1 2 2 2
  spline S25 degree 2 poles (12.2893, 9.7394) (12.1077, 9.5365) (11.6793, 9.4023) (11.4195, 9.4862) knots 0 0 0 1 2 2 2
  spline S26 degree 2 poles (11.4195, 9.4862) (11.1866, 9.5577) (10.6874, 9.9015) (10.4142, 10.1194) knots 0 0 0 1 2 2 2
  line L21 (10.4142, 10.1194) -> (10.3574, 10.0559)
  spline S27 degree 2 poles (10.3574, 10.0559) (10.2553, 9.9418) (10.1984, 9.7378) (10.2258, 9.6409) knots 0 0 0 1 2 2 2
  spline S28 degree 2 poles (10.2258, 9.6409) (10.2533, 9.544) (10.4124, 9.356) (10.5096, 9.269) knots 0 0 0 1 2 2 2
  spline S29 degree 2 poles (10.5096, 9.269) (10.6238, 9.1668) (10.9929, 8.9584) (11.2058, 8.8858) knots 0 0 0 1 2 2 2
  line L22 (11.2058, 8.8858) -> (11.2248, 8.8688)
  line L23 (11.2248, 8.8688) -> (10.9241, 8.5327)
  spline S30 degree 2 poles (10.9241, 8.5327) (10.8106, 8.5887) (10.4135, 8.8298) (10.2465, 8.9792) knots 0 0 0 1 2 2 2
  spline S31 degree 2 poles (10.2465, 8.9792) (10.0436, 9.1607) (9.8234, 9.4719) (9.7873, 9.6527) knots 0 0 0 1 2 2 2
  spline S32 degree 2 poles (9.7873, 9.6527) (9.7514, 9.8294) (9.8745, 10.1798) (10.039, 10.3637) knots 0 0 0 1 2 2 2
  line L24 (10.039, 10.3637) -> (11.2362, 11.7017)
  line L25 (11.2362, 11.7017) -> (11.5659, 11.4066)
  line L26 (11.5659, 11.4066) -> (11.3806, 11.1995)
  line L27 (11.1347, 10.9247) -> (10.6487, 10.3815)
  spline S33 degree 2 poles (10.6487, 10.3815) (10.7765, 10.2861) (11.1659, 10.0024) (11.3082, 9.936) knots 0 0 0 1 2 2 2
  spline S34 degree 2 poles (11.3082, 9.936) (11.4752, 9.8589) (11.7958, 9.8727) (11.9282, 10.0207) knots 0 0 0 1 2 2 2
  spline S35 degree 2 poles (11.9282, 10.0207) (12.0795, 10.1898) (12.0424, 10.5312) (11.8606, 10.6939) knots 0 0 0 1 2 2 2
  spline S36 degree 2 poles (11.8606, 10.6939) (11.7063, 10.8319) (11.3335, 10.9257) (11.1347, 10.9247) knots 0 0 0 1 2 2 2
  spline S37 degree 2 poles (10.2865, 12.6351) (10.483, 12.4593) (10.7288, 12.0491) (10.7879, 11.8897) knots 0 0 0 1 2 2 2
  line L28 (10.7879, 11.8897) -> (10.4569, 11.5198)
  line L29 (10.4569, 11.5198) -> (10.44, 11.5349)
  spline S38 degree 2 poles (10.44, 11.5349) (10.428, 11.6065) (10.3857, 11.789) (10.3303, 11.9185) knots 0 0 0 1 2 2 2
  spline S39 degree 2 poles (10.3303, 11.9185) (10.2838, 12.0324) (10.1338, 12.2731) (10.026, 12.3696) knots 0 0 0 1 2 2 2
  spline S40 degree 2 poles (10.026, 12.3696) (9.9478, 12.4396) (9.736, 12.5644) (9.6672, 12.5726) knots 0 0 0 1 2 2 2
  spline S41 degree 2 poles (9.6672, 12.5726) (9.57, 12.5873) (9.4337, 12.5456) (9.3505, 12.4526) knots 0 0 0 1 2 2 2
  spline S42 degree 2 poles (9.3505, 12.4526) (9.2465, 12.3363) (9.2655, 12.1024) (9.3923, 11.9166) knots 0 0 0 1 2 2 2
  spline S43 degree 2 poles (9.3923, 11.9166) (9.4425, 11.8451) (9.6076, 11.6212) (9.6735, 11.5204) knots 0 0 0 1 2 2 2
  spline S44 degree 2 poles (9.6735, 11.5204) (9.8389, 11.2544) (9.7997, 10.8023) (9.6276, 10.61) knots 0 0 0 1 2 2 2
  spline S45 degree 2 poles (9.6276, 10.61) (9.3893, 10.3436) (8.6929, 10.3692) (8.3632, 10.6643) knots 0 0 0 1 2 2 2
  spline S46 degree 2 poles (8.3632, 10.6643) (8.2004, 10.8099) (7.9426, 11.1852) (7.8854, 11.3468) knots 0 0 0 1 2 2 2
  line L30 (7.8854, 11.3468) -> (8.2012, 11.6998)
  line L31 (8.2012, 11.6998) -> (8.2181, 11.6846)
  spline S47 degree 2 poles (8.2181, 11.6846) (8.2542, 11.4697) (8.4587, 11.0773) (8.6173, 10.9355) knots 0 0 0 1 2 2 2
  spline S48 degree 2 poles (8.6173, 10.9355) (8.78, 10.7899) (9.127, 10.7268) (9.25, 10.8642) knots 0 0 0 1 2 2 2
  spline S49 degree 2 poles (9.25, 10.8642) (9.3615, 10.9889) (9.3362, 11.2285) (9.2222, 11.3989) knots 0 0 0 1 2 2 2
  spline S50 degree 2 poles (9.2222, 11.3989) (9.1674, 11.4823) (9.0197, 11.683) (8.9411, 11.7951) knots 0 0 0 1 2 2 2
  spline S51 degree 2 poles (8.9411, 11.7951) (8.7747, 12.043) (8.7799, 12.4912) (8.9747, 12.7089) knots 0 0 0 1 2 2 2
  spline S52 degree 2 poles (8.9747, 12.7089) (9.0882, 12.8357) (9.388, 12.9709) (9.559, 12.9663) knots 0 0 0 1 2 2 2
  spline S53 degree 2 poles (9.559, 12.9663) (9.7401, 12.9603) (10.0856, 12.8148) (10.2865, 12.6351) knots 0 0 0 1 2 2 2
  spline S54 degree 2 poles (8.3632, 14.3522) (8.8324, 13.9323) (8.8773, 12.9445) (8.4423, 12.4584) knots 0 0 0 1 2 2 2
  spline S55 degree 2 poles (8.4423, 12.4584) (8.0149, 11.9807) (7.0071, 11.8624) (6.6033, 12.2236) knots 0 0 0 1 2 2 2
  spline S56 degree 2 poles (6.6033, 12.2236) (6.4216, 12.3863) (6.235, 12.7435) (6.2316, 12.9482) knots 0 0 0 1 2 2 2
  spline S57 degree 2 poles (6.2316, 12.9482) (6.2262, 13.1548) (6.4035, 13.5784) (6.6135, 13.813) knots 0 0 0 1 2 2 2
  line L32 (6.6135, 13.813) -> (6.7742, 13.9927)
  line L33 (6.7742, 13.9927) -> (8.1291, 12.7804)
  spline S58 degree 2 poles (8.1291, 12.7804) (8.4336, 13.1207) (8.4146, 13.7886) (8.1102, 14.0609) knots 0 0 0 1 2 2 2
  spline S59 degree 2 poles (8.1102, 14.0609) (8.0024, 14.1574) (7.7496, 14.296) (7.631, 14.3336) knots 0 0 0 1 2 2 2
  spline S60 degree 2 poles (7.631, 14.3336) (7.5044, 14.3707) (7.3157, 14.4064) (7.2452, 14.4086) knots 0 0 0 1 2 2 2
  line L34 (7.2452, 14.4086) -> (7.2262, 14.4256)
  line L35 (7.2262, 14.4256) -> (7.5477, 14.7849)
  spline S61 degree 2 poles (7.5477, 14.7849) (7.6256, 14.7571) (7.8594, 14.6697) (7.9441, 14.6282) knots 0 0 0 1 2 2 2
  spline S62 degree 2 poles (7.9441, 14.6282) (8.0638, 14.5705) (8.2448, 14.4581) (8.3632, 14.3522) knots 0 0 0 1 2 2 2
  spline S63 degree 2 poles (6.8704, 13.4537) (6.7555, 13.3168) (6.6365, 13.0731) (6.6307, 12.9603) knots 0 0 0 1 2 2 2
  spline S64 degree 2 poles (6.6307, 12.9603) (6.6216, 12.8353) (6.7313, 12.5963) (6.8644, 12.4772) knots 0 0 0 1 2 2 2
  spline S65 degree 2 poles (6.8644, 12.4772) (6.9955, 12.3599) (7.2494, 12.2736) (7.3935, 12.2816) knots 0 0 0 1 2 2 2
  spline S66 degree 2 poles (7.3935, 12.2816) (7.5375, 12.2936) (7.7819, 12.4136) (7.9041, 12.5289) knots 0 0 0 1 2 2 2
  line L36 (7.9041, 12.5289) -> (6.8704, 13.4537)
  line L37 (2.0032, 15.2663) -> (4.9922, 17.2883)
  line L38 (4.9922, 17.2883) -> (5.3811, 16.9404)
  line L39 (5.3811, 16.9404) -> (3.9751, 14.3012)
  line L40 (3.9751, 14.3012) -> (6.4274, 16.0042)
  line L41 (6.4274, 16.0042) -> (6.8121, 15.66)
  line L42 (6.8121, 15.66) -> (5.1442, 12.4559)
  line L43 (5.1442, 12.4559) -> (4.787, 12.7755)
  line L44 (4.787, 12.7755) -> (6.1975, 15.4069)
  line L45 (6.1975, 15.4069) -> (3.7428, 13.7098)
  line L46 (3.7428, 13.7098) -> (3.3898, 14.0256)
  line L47 (3.3898, 14.0256) -> (4.823, 16.6824)
  line L48 (4.823, 16.6824) -> (2.3435, 14.9618)
  line L49 (2.3435, 14.9618) -> (2.0032, 15.2663)
  spline S67 degree 2 poles (1.5674, 18.5905) (2.01, 19.0851) (2.9678, 19.1986) (3.3652, 18.843) knots 0 0 0 1 2 2 2
  spline S68 degree 2 poles (3.3652, 18.843) (3.7731, 18.478) (3.7429, 17.5042) (3.3155, 17.0265) knots 0 0 0 1 2 2 2
  spline S69 degree 2 poles (3.3155, 17.0265) (2.8767, 16.5361) (1.9087, 16.424) (1.5156, 16.7758) knots 0 0 0 1 2 2 2
  spline S70 degree 2 poles (1.5156, 16.7758) (1.1182, 17.1314) (1.1267, 18.098) (1.5674, 18.5905) knots 0 0 0 1 2 2 2
  spline S71 degree 2 poles (1.9077, 18.286) (1.5673, 17.9055) (1.5132, 17.2879) (1.769, 17.059) knots 0 0 0 1 2 2 2
  spline S72 degree 2 poles (1.769, 17.059) (2.0248, 16.8302) (2.6347, 16.9505) (2.9752, 17.3309) knots 0 0 0 1 2 2 2
  spline S73 degree 2 poles (2.9752, 17.3309) (3.3061, 17.7008) (3.3675, 18.331) (3.1118, 18.5598) knots 0 0 0 1 2 2 2
  spline S74 degree 2 poles (3.1118, 18.5598) (2.8581, 18.7867) (2.2444, 18.6623) (1.9077, 18.286) knots 0 0 0 1 2 2 2
  line L50 (-0.3684, 19.196) -> (-0.3515, 19.1809)
  spline S75 degree 2 poles (-0.3515, 19.1809) (-0.3229, 19.1363) (-0.2443, 19.0583) (-0.1872, 19.0072) knots 0 0 0 1 2 2 2
  spline S76 degree 2 poles (-0.1872, 19.0072) (-0.0541, 18.8881) (0.3121, 18.7698) (0.5326, 18.7781) knots 0 0 0 1 2 2 2
  line L51 (0.5326, 18.7781) -> (1.7751, 20.1668)
  line L52 (1.7751, 20.1668) -> (2.1048, 19.8718)
  line L53 (2.1048, 19.8718) -> (0.3536, 17.9144)
  line L54 (0.3536, 17.9144) -> (0.0238, 18.2095)
  line L55 (0.0238, 18.2095) -> (0.2848, 18.5012)
  spline S77 degree 2 poles (0.2848, 18.5012) (-0.0386, 18.5013) (-0.4243, 18.6104) (-0.5511, 18.7239) knots 0 0 0 1 2 2 2
  spline S78 degree 2 poles (-0.5511, 18.7239) (-0.6018, 18.7693) (-0.6488, 18.8189) (-0.6748, 18.8536) knots 0 0 0 1 2 2 2
  line L56 (-0.6748, 18.8536) -> (-0.3684, 19.196)
  line L57 (-0.81, 22.4798) -> (-0.3767, 22.0921)
  line L58 (-0.3767, 22.0921) -> (-0.4949, 20.4966)
  line L59 (-0.4949, 20.4966) -> (-0.2504, 20.5062)
  line L60 (-0.2504, 20.5062) -> (0.4815, 21.3242)
  line L61 (0.4815, 21.3242) -> (0.8112, 21.0292)
  line L62 (0.8112, 21.0292) -> (-1.6266, 18.3046)
  line L63 (-1.6266, 18.3046) -> (-1.9563, 18.5996)
  line L64 (-1.9563, 18.5996) -> (-0.5303, 20.1934)
  line L65 (-0.5303, 20.1934) -> (-2.0434, 20.0591)
  line L66 (-2.0434, 20.0591) -> (-2.4535, 20.426)
  line L67 (-2.4535, 20.426) -> (-0.9184, 20.5253)
  line L68 (-0.9184, 20.5253) -> (-0.81, 22.4798)
  line L69 (-1.4864, 23.085) -> (-1.0679, 22.7105)
  line L70 (-1.0679, 22.7105) -> (-1.5142, 22.2116)
  line L71 (-1.5142, 22.2116) -> (-1.9327, 22.5861)
  line L72 (-1.9327, 22.5861) -> (-1.4864, 23.085)
  line L73 (-2.9956, 24.4353) -> (-1.9852, 23.5313)
  line L74 (-1.9852, 23.5313) -> (-2.2235, 23.265)
  line L75 (-2.2235, 23.265) -> (-2.5554, 23.5619)
  line L76 (-2.5554, 23.5619) -> (-4.4126, 21.4862)
  line L77 (-4.4126, 21.4862) -> (-4.0807, 21.1893)
  line L78 (-4.0807, 21.1893) -> (-4.319, 20.9229)
  line L79 (-4.319, 20.9229) -> (-5.3294, 21.8269)
  line L80 (-5.3294, 21.8269) -> (-5.0911, 22.0933)
  line L81 (-5.0911, 22.0933) -> (-4.7592, 21.7963)
  line L82 (-4.7592, 21.7963) -> (-2.902, 23.872)
  line L83 (-2.902, 23.872) -> (-3.2339, 24.169)
  line L84 (-3.2339, 24.169) -> (-2.9956, 24.4353)
  line L85 (-3.1436, 24.5677) -> (-6.3567, 22.7461)
  line L86 (-6.3567, 22.7461) -> (-6.7836, 23.1281)
  line L87 (-6.7836, 23.1281) -> (-5.3292, 26.5232)
  line L88 (-5.3292, 26.5232) -> (-4.9635, 26.196)
  line L89 (-4.9635, 26.196) -> (-5.3792, 25.255)
  line L90 (-5.3792, 25.255) -> (-4.3837, 24.3642)
  line L91 (-4.3837, 24.3642) -> (-3.4944, 24.8816)
  line L92 (-3.4944, 24.8816) -> (-3.1436, 24.5677)
  line L93 (-5.5489, 24.8739) -> (-6.244, 23.2846)
  line L94 (-6.244, 23.2846) -> (-4.7435, 24.1534)
  line L95 (-4.7435, 24.1534) -> (-5.5489, 24.8739)
  line L96 (-5.2953, 26.4929) -> (-8.5084, 24.6713)
  line L97 (-8.5084, 24.6713) -> (-8.9354, 25.0534)
  line L98 (-8.9354, 25.0534) -> (-7.481, 28.4485)
  line L99 (-7.481, 28.4485) -> (-7.1153, 28.1213)
  line L100 (-7.1153, 28.1213) -> (-7.531, 27.1802)
  line L101 (-7.531, 27.1802) -> (-6.5354, 26.2895)
  line L102 (-6.5354, 26.2895) -> (-5.6462, 26.8069)
  line L103 (-5.6462, 26.8069) -> (-5.2953, 26.4929)
  line L104 (-7.7007, 26.7992) -> (-8.3957, 25.2099)
  line L105 (-8.3957, 25.2099) -> (-6.8953, 26.0786)
  line L106 (-6.8953, 26.0786) -> (-7.7007, 26.7992)
  line L107 (-9.9646, 30.6707) -> (-9.6179, 30.3605)
  line L108 (-9.6179, 30.3605) -> (-11.6283, 28.1136)
  line L109 (-11.6283, 28.1136) -> (-9.5803, 29.0329)
  line L110 (-9.5803, 29.0329) -> (-9.369, 28.8437)
  line L111 (-9.369, 28.8437) -> (-10.062, 26.7122)
  line L112 (-10.062, 26.7122) -> (-8.0517, 28.9591)
  line L113 (-8.0517, 28.9591) -> (-7.7283, 28.6697)
  line L114 (-7.7283, 28.6697) -> (-10.062, 26.0614)
  line L115 (-10.062, 26.0614) -> (-10.5355, 26.485)
  line L116 (-10.5355, 26.485) -> (-9.8873, 28.5197)
  line L117 (-9.8873, 28.5197) -> (-11.8164, 27.6311)
  line L118 (-11.8164, 27.6311) -> (-12.2984, 28.0623)
  line L119 (-12.2984, 28.0623) -> (-9.9646, 30.6707)
  point P0 (21.1, 0)
  constraints: 2 other
emboss "Emboss1" sketch "Sketch26" operation cut depth 1 direction (0, 0, 1)
body "Solid1"
body "Srf1"
